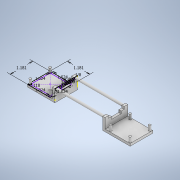
# Autodesk Inventor part: CDSAXS-Capillary-Frame-For2Sensors
Saved by Autodesk Inventor 2020 (Build 240168000, 168)
## iProperties
Created: 2023-02-02
Part Number: CDSAXS-Capillary-Frame-For2Sensors
Material: Generic
Document SubType Name: Modeling
Designer: Beaucage
Density: 1 g/cm^3
Appearance: Default
Author: Beaucage
Autodesk Inventor part; units mm, degrees
ref_plane "YZ Plane" through (0, 0, 0) normal (1, 0, 0) x (0, 1, 0)
ref_plane "XZ Plane" through (0, 0, 0) normal (0, 1, 0) x (-1, 0, 0)
ref_plane "XY Plane" through (0, 0, 0) normal (0, 0, 1) x (1, 0, 0)
sketch "Sketch1" plane through (0, 0, 0) normal (0, 1, 0) x (-1, 0, 0)
  line L0 (0, 0) -> (30, 0)
  line L1 (30, 0) -> (30, -30)
  line L2 (30, -30) -> (0, -30)
  line L3 (0, -30) -> (0, 0)
  line L4 (28, -2) -> (2, -2)
  line L5 (2, -2) -> (2, -28)
  line L6 (2, -28) -> (28, -28)
  line L7 (28, -28) -> (28, -2)
  line L8 (28, -2) -> (2, -28) construction
  line L9 (2, -2) -> (28, -28) construction
  circle A0 centre (28, -2) radius 1.5
  circle A1 centre (28, -28) radius 1.5
  circle A2 centre (2, -2) radius 1.5
  circle A3 centre (2, -28) radius 1.5
  point P0 (15, -15)
  dimension "d0" = 30
  dimension "d1" = 30
  dimension "d2" = 26
  dimension "d3" = 26
  dimension "d4" = 3
  dimension "d7" = 26
  dimension "d10" = 26
  constraints: 20 end point, 4 centre point, 4 parallel, 3 horizontal, 2 midpoint, 2 perpendicular, 1 coincident, 1 vertical, 6 other
  measures "d0" distance of L1.end L2.end
  measures "d1" distance of L0.end L1.end
  measures "d2" distance of L6.end L5.end
  measures "d3" distance of L5.end L4.end
  measures "d4" diameter of A0
  measures "d7" distance of A0.centre A1.centre
  measures "d10" distance of A0.centre A2.centre
extrude "Extrusion1" add sketch "Sketch1" against normal blind 3.175 contours L0 L1 L2 L3 | A2 L5 L4 | L4 L5 A2 | L4 A0 L7 A1 L6 A3 L5 A2 | A0 L7 L4 | L4 L7 A0 | A3 L6 L5 | L5 L6 A3 | A1 L6 L7 | L7 L6 A1
extrude "Extrusion2" add sketch "Sketch1" along normal blind 6.35 contours A2 L5 L4 | L4 L5 A2 | A0 L7 L4 | L4 L7 A0 | A3 L6 L5 | L5 L6 A3 | A1 L6 L7 | L7 L6 A1
sketch "Sketch2" plane through (0, 0, 0) normal (1, 0, 0) x (0, 0, -1)
  line L0 (0, 0) -> (0, -3.175) projected
  line L1 (0, 0) -> (30, 0) projected
  line L2 (0, -3.175) -> (30, -3.175)
  line L3 (30, -3.175) -> (30, 0)
  line L4 (30, 0) -> (0, 0)
  line L5 (0, 0) -> (0, -3.175)
  constraints: 8 end point, 2 parallel, 1 horizontal, 1 perpendicular
extrude "Extrusion3" add sketch "Sketch2" along normal blind 6.35
sketch "Sketch3" plane through (0, 0, 0) normal (0, 1, 0) x (1, 0, 0)
  line L0 (6.35, 0) -> (6.35, 30) projected
  line L1 (-30, 30) -> (6.35, 30) projected
  line L2 (6.35, 0) -> (3.175, 0)
  line L3 (3.175, 0) -> (3.175, 30)
  line L4 (3.175, 30) -> (6.35, 30)
  line L5 (6.35, 30) -> (6.35, 0)
  point P0 (0, 0)
  dimension "d19" = 3.175
  constraints: 8 end point, 2 parallel, 1 horizontal, 1 perpendicular, 1 point on line
  measures "d19" distance of L3.end L4.end
extrude "Extrusion4" add sketch "Sketch3" along normal blind 13.175
sketch "Sketch4" plane through (6.35, 0, 0) normal (1, 0, 0) x (0, 0, -1)
  line L0 (30, 13.175) -> (0, 13.175) projected
  line L1 (30, 0) -> (30, 13.175) projected
  line L2 (0, 13.175) -> (30, 13.175)
  line L3 (15, 13.175) -> (15, 11.5875)
  line L4 (15, 11.5875) -> (27.7, 11.5875)
  line L5 (27.7, 11.5875) -> (2.3, 11.5875)
  circle A0 centre (2.3, 11.5875) radius 1.5875
  circle A1 centre (27.7, 11.5875) radius 1.5875
  line L6 (4.7076, 10) -> (25.2924, 10)
  line L7 (25.2924, 10) -> (25.2924, 13.175)
  line L8 (25.2924, 13.175) -> (4.7076, 13.175)
  line L9 (4.7076, 13.175) -> (4.7076, 10)
  line L10 (4.7076, 10) -> (25.2924, 13.175) construction
  line L11 (25.2924, 10) -> (4.7076, 13.175) construction
  line L12 (8.65, 6.825) -> (21.35, 6.825)
  line L13 (21.35, 6.825) -> (21.35, 13.175)
  line L14 (21.35, 13.175) -> (8.65, 13.175)
  line L15 (8.65, 13.175) -> (8.65, 6.825)
  line L16 (8.65, 6.825) -> (21.35, 13.175) construction
  line L17 (21.35, 6.825) -> (8.65, 13.175) construction
  point P0 (0, 0)
  point P1 (15, 10)
  point P2 (21.35, 10)
  point P3 (8.65, 10)
  dimension "d22" = 1.5875
  dimension "d23" = 12.7
  dimension "d24" = 90
  dimension "d25" = 25.4
  dimension "d26" = 3.175
  dimension "d27" = 3.175
  constraints: 32 end point, 6 midpoint, 4 parallel, 4 perpendicular, 3 point on line, 2 centre point, 2 coincident, 2 horizontal, 1 vertical
  measures "d22" distance of L3.start L3.end
  measures "d23" distance of L3.end L4.end
  measures "d24" angle of L4 L3
  measures "d25" distance of L4.end L5.end
  measures "d26" diameter of A0
  measures "d27" diameter of A1
extrude "Extrusion5" add sketch "Sketch4" along normal blind 31.75 contours A1 | A0
extrude "Extrusion6" cut sketch "Sketch4" against normal blind 3.175 contours L7 L4 L13 L0 | L13 L4 L3 L0 | L7 L6 L13 L4 | L3 L5 L15 L0 | L13 L6 L15 L5 L4 | L15 L5 L9 L0 | L13 L12 L15 L6 | L15 L6 L9 L5
mirror "Mirror1" about plane through (38.1, 11.5875, -27.7) normal (1, 0, 0) of "Extrusion1", "Extrusion2", "Extrusion3", "Extrusion4", "Extrusion5", "Extrusion6"
body "Solid1"
